Autodesk Fusion 360 part; units mm, degrees
note: some values were not read from the file. Set by a fixed rule: the direction of a hole.
(part 4 of 4)
sketch "草图4" plane through (0, 0, 12) normal (0, 0, 1) x (-1, 0, 0)
  circle A0 centre (-30, 0) radius 1.25
  circle A1 centre (30, 0) radius 1.25
  arc A2 (-16.1674, -6.698) -> (16.1674, -6.698) centre (0, 0) ccw
  arc A3 (18.7154, -4.8546) -> (16.1674, -6.698) centre (18.939, -7.8463) ccw
  line L0 (18.7154, -4.8546) -> (30.2981, -3.9889)
  arc A4 (30.2981, -3.9889) -> (30.2981, 3.9889) centre (30, 0) ccw
  line L1 (30.2981, 3.9889) -> (18.7154, 4.8546)
  arc A5 (16.1674, 6.698) -> (18.7154, 4.8546) centre (18.939, 7.8463) ccw
  arc A6 (16.1674, 6.698) -> (-16.1674, 6.698) centre (0, 0) ccw
  arc A7 (-18.7154, 4.8546) -> (-16.1674, 6.698) centre (-18.939, 7.8463) ccw
  line L2 (-18.7154, 4.8546) -> (-30.2981, 3.9889)
  arc A8 (-30.2981, 3.9889) -> (-30.2981, -3.9889) centre (-30, 0) ccw
  line L3 (-30.2981, -3.9889) -> (-18.7154, -4.8546)
  arc A9 (-16.1674, -6.698) -> (-18.7154, -4.8546) centre (-18.939, -7.8463) ccw
  circle A10 centre (11.6913, 6.75) radius 3
  circle A11 centre (0, -13.5) radius 3
  circle A12 centre (-11.6913, -6.75) radius 3
  circle A13 centre (0, 13.5) radius 3
  circle A14 centre (11.6913, -6.75) radius 3
  circle A15 centre (-11.6913, 6.75) radius 3
  circle A16 centre (0, 0) radius 8
  dimension "d32" = 16
  constraint concentric A2 A16
  measures "d32" diameter of A16
extrude "拉伸7" cut sketch "草图4" against normal up to surface (12 mm away) contours A16 bodies 1

design "J4-J5-Out"
part number: 2026-08-07-17-32-29-090
Autodesk Fusion 360 part; units mm, degrees
sketch "草图1" plane through (0, 0, 0) normal (0, 0, 1) x (1, 0, 0)
  circle A0 centre (0, 0) radius 19
  circle A1 centre (0, 0) radius 25 construction
  arc A2 (-28.5, 0) -> (28.5, 0) centre (0, 0) ccw
  line L0 (-28.5, 0) -> (-28.5, 18)
  line L1 (-28.5, 18) -> (-33.5, 18)
  line L2 (-33.5, 18) -> (-33.5, 58)
  line L3 (-33.5, 58) -> (33.5, 58)
  line L4 (33.5, 58) -> (33.5, 18)
  line L5 (33.5, 18) -> (28.5, 18)
  line L6 (28.5, 18) -> (28.5, 0)
  line L7 (0, 0) -> (0, 58) construction
  circle A3 centre (-12.5, -21.6506) radius 1.6
  circle A4 centre (12.5, -21.6506) radius 1.6
  circle A5 centre (25, 0) radius 1.6
  circle A6 centre (12.5, 21.6506) radius 1.6
  circle A7 centre (-12.5, 21.6506) radius 1.6
  circle A8 centre (-25, 0) radius 1.6
  line L8 (-15, 46) -> (15, 46)
  line L9 (15, 46) -> (15, 33)
  line L10 (15, 33) -> (-15, 33)
  line L11 (-15, 33) -> (-15, 46)
  line L12 (-15, 46) -> (15, 33) construction
  line L13 (15, 46) -> (-15, 33) construction
  point P0 (0, 39.5)
  dimension "d1" = 28.5
  dimension "d2" = 50
  dimension "d3" = 38
  dimension "d4" = 3.2
  dimension "d6" = 360
  dimension "d7" = 67
  dimension "d8" = 40
  dimension "d9" = 58
  dimension "d10" = 13
  dimension "d12" = 30
  dimension "d104" = 12
  constraint coincident A0.centre A1.centre
  constraint concentric A0 A1
  constraint tangent A2 L0
  constraint vertical L0
  constraint perpendicular L0 L1
  constraint perpendicular L1 L2
  constraint perpendicular L2 L3
  constraint perpendicular L3 L4
  constraint perpendicular L4 L5
  constraint perpendicular L5 L6
  constraint tangent A2 L6
  constraint midpoint L3 L7.end
  constraint vertical L7
  constraint equal L2 L4
  constraint coincident A1 A3.centre
  constraint symmetric L7 A3.centre A4.centre
  constraint horizontal L8
  constraint perpendicular L8 L9
  constraint parallel L8 L10
  constraint parallel L9 L11
  constraint coincident L12 P0
  constraint coincident L13 P0
  constraint coincident L7 P0
  measures "d1" radius of A2
  measures "d2" diameter of A1
  measures "d3" diameter of A0
  measures "d4" diameter of A3
  measures "d7" distance of L2.end L3.end
  measures "d8" distance of L1.end L2.end
  measures "d9" distance of A0.centre L3
  measures "d10" distance of L8.start L10.end
  measures "d12" distance of L8.start L8.end
  measures "d104" distance of L3 L8
extrude "拉伸1" add sketch "草图1" along normal blind 5 makes body 1
hole "孔1" at (25, 0, 0) at (12.5, 21.6506, 0) at (-12.5, 21.6506, 0) at (-25, 0, 0) at (-12.5, -21.6506, 0) at (12.5, -21.6506, 0) direction (0, 0, 1) diameter 3.2 depth 10 tip angle 180 countersink diameter 6.3 countersink angle 90 bodies 1
sketch "草图5" plane through (0, 0, 0) normal (0, 0, -1) x (1, 0, 0)
  arc A0 (28.5, 0) -> (-28.5, 0) centre (0, 0) ccw
  line L0 (-28.5, 0) -> (-28.5, -18)
  line L1 (-28.5, -18) -> (-33.5, -18)
  line L2 (-33.5, -18) -> (-33.5, -58)
  line L3 (-33.5, -58) -> (33.5, -58)
  line L4 (33.5, -58) -> (33.5, -18)
  line L5 (33.5, -18) -> (28.5, -18)
  line L6 (28.5, -18) -> (28.5, 0)
  circle A1 centre (0, 0) radius 19
  line L7 (-15, -33) -> (15, -33)
  line L8 (15, -33) -> (15, -46)
  line L9 (15, -46) -> (-15, -46)
  line L10 (-15, -46) -> (-15, -33)
  line L11 (33.5, -18) -> (25.5, -18)
  line L12 (25.5, -18) -> (25.5, -58)
  line L13 (25.5, -58) -> (33.5, -58)
  line L14 (33.5, -58) -> (33.5, -18)
  line L15 (-33.5, -18) -> (-25.5, -18)
  line L16 (-25.5, -18) -> (-25.5, -58)
  line L17 (-25.5, -58) -> (-33.5, -58)
  line L18 (-33.5, -58) -> (-33.5, -18)
  circle A2 centre (12.5, 21.6506) radius 3.15
  circle A3 centre (-25, 0) radius 3.15
  circle A4 centre (12.5, -21.6506) radius 3.15
  circle A5 centre (25, 0) radius 3.15
  circle A6 centre (-12.5, -21.6506) radius 3.15
  circle A7 centre (-12.5, 21.6506) radius 3.15
  dimension "d29" = 8
  constraint horizontal L11
  constraint vertical L12
  constraint horizontal L13
  constraint vertical L14
  constraint coincident L3 L12.end
  constraint coincident L4.end L5.start
  constraint horizontal L15
  constraint vertical L16
  constraint horizontal L17
  constraint vertical L18
  constraint coincident L3 L16.end
  constraint coincident L1.end L2.start
  constraint equal L13 L17
  measures "d29" distance of L12.end L3.end
extrude "拉伸4" add sketch "草图5" along normal blind 3 contours L3 L4 L5 L11 L12 L13 L14 | L1 L2 L3 L15 L16 L17 L18 bodies 1
sketch "草图10" plane through (0, 0, 5) normal (0, 0, 1) x (-1, 0, 0)
  arc A0 (28.5, 0) -> (-28.5, 0) centre (0, 0) ccw
  line L0 (-28.5, 0) -> (-28.5, -18)
  line L1 (-28.5, -18) -> (-33.5, -18)
  line L2 (-33.5, -18) -> (-33.5, -58)
  line L3 (-33.5, -58) -> (33.5, -58)
  line L4 (33.5, -58) -> (33.5, -18)
  line L5 (33.5, -18) -> (28.5, -18)
  line L6 (28.5, -18) -> (28.5, 0)
  circle A1 centre (25, 0) radius 1.6
  line L7 (-15, -33) -> (15, -33)
  line L8 (15, -33) -> (15, -46)
  line L9 (15, -46) -> (-15, -46)
  line L10 (-15, -46) -> (-15, -33)
  circle A2 centre (12.5, -21.6506) radius 1.6
  circle A3 centre (-25, 0) radius 1.6
  circle A4 centre (-12.5, -21.6506) radius 1.6
  circle A5 centre (12.5, 21.6506) radius 1.6
  circle A6 centre (-12.5, 21.6506) radius 1.6
  circle A7 centre (0, 0) radius 19
  line L11 (-20, -33) -> (20, -33) construction
  line L12 (0, 0) -> (0, -33) construction
  circle A8 centre (-20, -33) radius 1.6
  circle A9 centre (20, -33) radius 1.6
  dimension "d78" = 3.2
  dimension "d79" = 40
  dimension "d80" = 33
  constraint perpendicular L8 L11
  constraint coincident A0.centre A7.centre
  constraint midpoint L11 L12.end
  constraint vertical L12
  constraint coincident L11.start A8.centre
  constraint coincident L11.end A9.centre
  constraint equal A8 A9
  measures "d78" diameter of A8
  measures "d79" distance of L11.start L11.end
  measures "d80" distance of A0.centre L12.end
extrude "拉伸10" cut sketch "草图10" against normal up to surface (5 mm away) contours A8 | A9 bodies 1
sketch "草图12" plane through (0, 0, 5) normal (0, 0, 1) x (-1, 0, 0)
  circle A0 centre (-25, 0) radius 1.6
  circle A1 centre (-12.5, 21.6506) radius 1.6
  circle A2 centre (-12.5, -21.6506) radius 1.6
  line L0 (-15, -33) -> (15, -33)
  line L1 (15, -33) -> (15, -46)
  line L2 (15, -46) -> (-15, -46)
  line L3 (-15, -46) -> (-15, -33)
  circle A3 centre (25, 0) radius 1.6
  circle A4 centre (12.5, 21.6506) radius 1.6
  circle A5 centre (12.5, -21.6506) radius 1.6
  circle A6 centre (0, 0) radius 19
  arc A7 (28.5, 0) -> (-28.5, 0) centre (0, 0) ccw
  line L4 (-28.5, 0) -> (-28.5, -18)
  line L5 (-33.5, -18) -> (-33.5, -58)
  line L6 (-33.5, -58) -> (33.5, -58)
  line L7 (33.5, -58) -> (33.5, -18)
  line L8 (28.5, -18) -> (28.5, 0)
  circle A8 centre (20, -33) radius 1.6
  circle A9 centre (-20, -33) radius 1.6
  line L9 (-24, -58) -> (-15, -50)
  line L10 (15, -50) -> (24, -58)
  line L11 (0, 0) -> (0, -58) construction
  line L12 (-15, -50) -> (15, -50)
  line L13 (-28.5, -18) -> (-33.5, -18)
  line L14 (33.5, -18) -> (28.5, -18)
  dimension "d96" = 48
  dimension "d106" = 8
  constraint coincident L6 L9.start
  constraint coincident L3 L9.end
  constraint coincident L1 L10.start
  constraint coincident L6 L10.end
  constraint coincident A6.centre A7.centre
  constraint midpoint L6 L11.end
  constraint symmetric L9.end L10.start L11
  constraint symmetric L9.start L10.end L11
  measures "d96" distance of L9.start L10.end
  measures "d106" distance of L6 L12
extrude "拉伸12" cut sketch "草图12" against normal up to surface (5 mm away) contours L6 L9 L10 L12 bodies 1
fillet "圆角5" radius 2.5 2 edges at (-24, 58, 2.5) (24, 58, 2.5) on bodies 1
fillet "圆角5" radius 3 2 edges at (15, 50, 2.5) (-15, 50, 2.5) on bodies 1
sketch "草图6" plane through (33.5, 0, 0) normal (1, 0, 0) x (0, 1, 0)
  line L0 (58, -3) -> (58, 5)
  line L1 (58, 5) -> (18, 5)
  line L2 (18, 5) -> (18, -3)
  line L3 (18, -3) -> (58, -3)
  line L4 (18, 1) -> (58, 1) construction
  line L5 (38, 5) -> (38, -3) construction
  circle A0 centre (22, 1) radius 1.25
  circle A1 centre (38, 1) radius 1.25
  circle A2 centre (54, 1) radius 1.25
  dimension "d32" = 2.5
  dimension "d33" = 32
  constraint midpoint L2 L4.start
  constraint midpoint L0 L4.end
  constraint coincident L1 L5.start
  constraint coincident L3 L5.end
  constraint perpendicular L3 L5
  constraint midpoint L1 L5.start
  constraint coincident L4 A0.centre
  constraint midpoint L5 A1.centre
  constraint coincident L4 A2.centre
  constraint equal A0 A1
  constraint equal A1 A2
  constraint symmetric L5 A0.centre A2.centre
  measures "d32" diameter of A0
  measures "d33" distance of A0.centre A2.centre
extrude "拉伸5" cut sketch "草图6" against normal blind 6 contours A0 | A1 | A2 bodies 1
mirror "镜像1" about plane through (0, 0, 0) normal (1, 0, 0) of "拉伸5"
fillet "圆角3" radius 5 2 edges at (28.5, 18, 2.5) (-28.5, 18, 2.5) on bodies 1
fillet "圆角3" radius 2 4 edges at (-15, 46, 2.5) (15, 46, 2.5) (15, 33, 2.5) (-15, 33, 2.5) on bodies 1
sketch "草图7" plane through (33.5, 0, 0) normal (1, 0, 0) x (0, 1, 0)
  circle A0 centre (22, 1) radius 1.25
  circle A1 centre (38, 1) radius 1.25
  circle A2 centre (54, 1) radius 1.25
  line L0 (18, 0) -> (18, -3)
  line L1 (18, -3) -> (58, -3)
  circle A3 centre (74, -41) radius 7
  circle A4 centre (74, -41) radius 13.5 construction
  circle A5 centre (63.75, -49.7857) radius 1.6
  line L2 (18, 0) -> (18, -3)
  arc A6 (54.0752, -39.2667) -> (75.3344, -21.0446) centre (74, -41) ccw
  line L3 (74, -41) -> (38, 1) construction
  line L4 (30, -11.1789) -> (54.0752, -39.2667)
  line L5 (75.3344, -21.0446) -> (58, -0.8211)
  circle A7 centre (76.4836, -54.2696) radius 1.6
  circle A8 centre (86.7336, -45.4839) radius 1.6
  circle A9 centre (84.25, -32.2143) radius 1.6
  circle A10 centre (71.5164, -27.7304) radius 1.6
  circle A11 centre (61.2664, -36.5161) radius 1.6
  circle A12 centre (22, 1) radius 1.6
  circle A13 centre (38, 1) radius 1.6
  circle A14 centre (54, 1) radius 1.6
  line L6 (58, 5) -> (18, 5)
  line L7 (58, -3) -> (58, 5)
  line L8 (30, -11.1789) -> (30, -3)
  line L9 (18, -3) -> (30, -3)
  line L10 (18, 5) -> (18, 0)
  dimension "d36" = 41
  dimension "d37" = 74
  dimension "d38" = 27
  dimension "d39" = 14
  dimension "d40" = 3.2
  dimension "d41" = 20
  dimension "d42" = 28
  dimension "d45" = 360
  dimension "d46" = 3.2
  dimension "d77" = 12
  constraint concentric A3 A4
  constraint coincident A4 A5.centre
  constraint coincident L0.start L2.start
  constraint coincident L0.end L1.start
  constraint coincident A3.centre A4.centre
  constraint coincident A1.centre L3.end
  constraint symmetric A6.start A6.end L3
  constraint parallel L4 L5
  constraint parallel L3 L4
  constraint symmetric L3 A10.centre A11.centre
  constraint concentric A0 A12
  constraint concentric A2 A14
  constraint equal A12 A13
  constraint equal A13 A14
  constraint coincident L1 L8.end
  constraint perpendicular L1 L8
  constraint coincident L5.end L7
  measures "d36" vertical distance of origin A3.centre
  measures "d37" horizontal distance of origin A3.centre
  measures "d38" diameter of A4
  measures "d39" diameter of A3
  measures "d40" diameter of A5
  measures "d41" radius of A6
  measures "d42" distance of L4 L5
  measures "d46" diameter of A12
  measures "d77" distance of L2 L8
extrude "拉伸6" add sketch "草图7" along normal blind 4 separate body contours L0 L1 L2 L6 L7 L9 L10 | L1 A6 L4 L5 L7 L8 | A5 | A7 | A8 | A9 | A10 | A11 makes body 2
sketch "草图8" plane through (37.5, 0, 0) normal (1, 0, 0) x (0, 1, 0)
  line L0 (58, -0.8211) -> (58, 5)
  line L1 (54.3615, -9) -> (65.6291, -22.2707)
  line L2 (65.6291, -22.2707) -> (56.4816, -30.0375)
  line L3 (56.4816, -30.0375) -> (38.6196, -9)
  line L4 (74, -41.4) -> (61.0554, -26.1541) construction
  line L5 (54.3615, -9) -> (38.6196, -9)
  line L6 (18, -3) -> (30, -3)
  circle A0 centre (74, -41) radius 7
  arc A1 (54.0752, -39.2667) -> (75.3344, -21.0446) centre (74, -41) ccw
  line L7 (75.3344, -21.0446) -> (58, -0.8211)
  line L8 (30, -3) -> (30, -11.1789)
  line L9 (30, -11.1789) -> (54.0752, -39.2667)
  circle A2 centre (38, 1) radius 1.6
  circle A3 centre (22, 1) radius 1.6
  circle A4 centre (54, 1) radius 1.6
  line L10 (58, 5) -> (18, 5)
  line L11 (18, 5) -> (18, -3)
  dimension "d51" = 20
  dimension "d53" = 12
  constraint perpendicular L1 L2
  constraint perpendicular L2 L3
  constraint midpoint L2 L4.end
  constraint horizontal L5
  measures "d51" distance of L2 L4.start
  measures "d53" distance of L1.end L2.end
extrude "拉伸7" cut sketch "草图8" against normal up to surface (4 mm away) contours L1 L2 L3 L5 bodies 2
fillet "圆角2" radius 2 4 edges at (35.5, 38.6196, -9) (35.5, 65.6291, -22.2707) (35.5, 56.4816, -30.0375) (35.5, 30, -3) on bodies 2
fillet "圆角2" radius 8 2 edges at (35.5, 54.3615, -9) (35.5, 58, -0.8211) on bodies 2
fillet "圆角2" radius 8 3 edges at (35.5, 75.3344, -21.0446) (35.5, 54.0752, -39.2667) (35.5, 30, -11.1789) on bodies 2
fillet "圆角2" radius 0.8 3 edges at (35.5, 18, 5) (35.5, 18, -3) (35.5, 58, 5) on bodies 2
mirror "镜像2" about plane through (0, 0, 0) normal (1, 0, 0) of "拉伸6", "拉伸7", "圆角2" makes body 3
extrude "拉伸8" cut sketch "草图7" along normal up to surface (4 mm away) contours A5 | A7 | A8 | A9 | A10 | A11 bodies 2
sketch "草图9" plane through (-37.5, 0, 0) normal (-1, 0, 0) x (0, -1, 0)
  line L0 (-74, -41.4) -> (-86.9446, -56.6459) construction
  circle A0 centre (-74, -41.4) radius 13 construction
  circle A1 centre (-86.2416, -45.7752) radius 1.6
  circle A2 centre (-76.3318, -54.1892) radius 1.6
  circle A3 centre (-64.0902, -49.814) radius 1.6
  circle A4 centre (-61.7584, -37.0248) radius 1.6
  circle A5 centre (-71.6682, -28.6108) radius 1.6
  circle A6 centre (-83.9098, -32.986) radius 1.6
  line L1 (-28, -3) -> (-18.8, -3)
  arc A7 (-31.9259, -13.4259) -> (-30, -8.2195) centre (-38, -8.2195) ccw
  line L2 (-30, -8.2195) -> (-30, -5)
  arc A8 (-28, -3) -> (-30, -5) centre (-28, -5) ccw
  arc A9 (-59.9259, -3.068) -> (-58, 2.1383) centre (-66, 2.1383) ccw
  line L3 (-59.9259, -3.068) -> (-73.3576, -18.7382)
  arc A10 (-77.8797, -21.3799) -> (-73.3576, -18.7382) centre (-79.4316, -13.5319) ccw
  arc A11 (-77.8797, -21.3799) -> (-54.0174, -41.8334) centre (-74, -41) ccw
  arc A12 (-52.0984, -36.9604) -> (-54.0174, -41.8334) centre (-46.0243, -42.1667) ccw
  line L4 (-52.0984, -36.9604) -> (-31.9259, -13.4259)
  line L5 (-58.0062, -28.743) -> (-64.1046, -23.5652)
  arc A13 (-64.3347, -20.7461) -> (-64.1046, -23.5652) centre (-62.8101, -22.0406) ccw
  line L6 (-64.3347, -20.7461) -> (-56.7577, -11.8222)
  arc A14 (-50.6594, -9) -> (-56.7577, -11.8222) centre (-50.6594, -17) ccw
  line L7 (-50.6594, -9) -> (-42.9414, -9)
  arc A15 (-41.4168, -12.2945) -> (-42.9414, -9) centre (-42.9414, -11) ccw
  line L8 (-41.4168, -12.2945) -> (-55.1872, -28.5129)
  arc A16 (-58.0062, -28.743) -> (-55.1872, -28.5129) centre (-56.7117, -27.2185) ccw
  circle A17 centre (-74, -41) radius 7
  line L9 (-18, -2.2) -> (-18, 4.2)
  line L10 (-18.8, 5) -> (-57.2, 5)
  line L11 (-58, 4.2) -> (-58, 2.1383)
  circle A18 centre (-54, 1) radius 1.6
  circle A19 centre (-22, 1) radius 1.6
  circle A20 centre (-38, 1) radius 1.6
  arc A21 (-18.8, -3) -> (-18, -2.2) centre (-18.8, -2.2) ccw
  arc A22 (-18, 4.2) -> (-18.8, 5) centre (-18.8, 4.2) ccw
  arc A23 (-57.2, 5) -> (-58, 4.2) centre (-57.2, 4.2) ccw
  dimension "d67" = 3.2
  dimension "d69" = 360
  dimension "d70" = 26
  constraint coincident L0.start A0.centre
  constraint coincident A0 A1.centre
  constraint symmetric L0 A1.centre A2.centre
  measures "d67" diameter of A1
  measures "d70" diameter of A0
extrude "拉伸9" cut sketch "草图9" against normal up to surface (4 mm away) contours A1 | A2 | A3 | A4 | A5 | A6 bodies 3
sketch "草图11" plane through (0, 0, 0) normal (0, 0, -1) x (1, 0, 0)
  circle A0 centre (0, 0) radius 19
  arc A1 (15, -35) -> (13, -33) centre (13, -35) ccw
  line L0 (15, -35) -> (15, -44)
  arc A2 (13, -46) -> (15, -44) centre (13, -44) ccw
  line L1 (13, -46) -> (-13, -46)
  arc A3 (-15, -44) -> (-13, -46) centre (-13, -44) ccw
  line L2 (-15, -44) -> (-15, -35)
  arc A4 (-13, -33) -> (-15, -35) centre (-13, -35) ccw
  line L3 (-13, -33) -> (13, -33)
  line L4 (-33.5, -18) -> (-25.5, -18)
  line L5 (-25.5, -18) -> (-25.5, -58)
  line L6 (24.9505, -58) -> (25.5, -58)
  line L7 (25.5, -58) -> (25.5, -18)
  line L8 (25.5, -18) -> (33.5, -18)
  arc A5 (28.5, -13) -> (33.5, -18) centre (33.5, -13) ccw
  line L9 (28.5, -13) -> (28.5, 0)
  arc A6 (28.5, 0) -> (-28.5, 0) centre (0, 0) ccw
  line L10 (-28.5, 0) -> (-28.5, -13)
  arc A7 (-33.5, -18) -> (-28.5, -13) centre (-33.5, -13) ccw
  circle A8 centre (-20, -33) radius 1.6
  circle A9 centre (20, -33) radius 1.6
  circle A10 centre (20, -33) radius 1.25
  circle A11 centre (-20, -33) radius 1.25
  line L11 (25, -28.5) -> (-25, -28.5)
  line L12 (-25, -28.5) -> (-25, -37.5)
  line L13 (-25, -37.5) -> (-15, -37.5)
  line L14 (-15, -37.5) -> (-15, -33)
  line L15 (-15, -33) -> (15, -33)
  line L16 (15, -33) -> (15, -37.5)
  line L17 (15, -37.5) -> (25, -37.5)
  line L18 (25, -37.5) -> (25, -28.5)
  line L19 (0, 0) -> (0, -28.5) construction
  line L20 (20, -33) -> (20, -37.5) construction
  circle A12 centre (-12.5, 21.6506) radius 3.15
  circle A13 centre (-12.5, -21.6506) radius 3.15
  circle A14 centre (25, 0) radius 3.15
  circle A15 centre (12.5, -21.6506) radius 3.15
  circle A16 centre (-25, 0) radius 3.15
  circle A17 centre (12.5, 21.6506) radius 3.15
  arc A18 (23.2896, -57.3685) -> (24.9505, -58) centre (24.9505, -55.5) ccw
  line L21 (-25.5, -58) -> (-24.9505, -58)
  arc A19 (-24.9505, -58) -> (-23.2896, -57.3685) centre (-24.9505, -55.5) ccw
  line L22 (-23.2896, -57.3685) -> (-15.8525, -50.7578)
  arc A20 (-13.8594, -50) -> (-15.8525, -50.7578) centre (-13.8594, -53) ccw
  line L23 (-13.8594, -50) -> (13.8594, -50)
  arc A21 (15.8525, -50.7578) -> (13.8594, -50) centre (13.8594, -53) ccw
  line L24 (15.8525, -50.7578) -> (23.2896, -57.3685)
  dimension "d83" = 2.5
  dimension "d84" = 4.5
  dimension "d85" = 10
  dimension "d86" = 9
  constraint concentric A9 A10
  constraint concentric A8 A11
  constraint equal A10 A11
  constraint horizontal L11
  constraint perpendicular L11 L12
  constraint perpendicular L12 L13
  constraint perpendicular L13 L14
  constraint perpendicular L14 L15
  constraint perpendicular L15 L16
  constraint perpendicular L16 L17
  constraint perpendicular L11 L18
  constraint midpoint L11 L19.end
  constraint vertical L19
  constraint coincident A0.centre A6.centre
  constraint symmetric L14.end L15.end L19
  constraint symmetric L12.end L17.end L19
  constraint coincident A9.centre A10.centre
  constraint midpoint L17 L20.end
  constraint vertical L20
  constraint collinear L3 L15
  measures "d83" diameter of A10
  measures "d84" distance of L3 L11
  measures "d85" distance of L16.end L17.end
  measures "d86" distance of L11.start L17.end
extrude "拉伸11" add sketch "草图11" along normal blind 8 separate body contours L0 L2 L3 L11 L12 L13 L14 L15 L16 L17 L18 | A8 | A9 makes body 4
fillet "圆角4" radius 2 8 edges at (15, 33, -4) (-15, 33, -4) (-15, 37.5, -4) (15, 37.5, -4) (25, 37.5, -4) (25, 28.5, -4) (-25, 28.5, -4) (-25, 37.5, -4) on bodies 4
equation "d1 = ( 57 / 2 ) * 1 mm"

design "yawτö╡µ£║σ¢║σ«Üµ¥┐"
part number: 2026-08-10-17-08-21-834
Autodesk Fusion 360 part; units mm, degrees
sketch "草图1" plane through (0, 0, 0) normal (0, 1, 0) x (1, 0, 0)
  circle A0 centre (0, 0) radius 20
  circle A1 centre (0, 0) radius 25 construction
  circle A2 centre (0, 25) radius 1.65
  circle A3 centre (-21.6506, 12.5) radius 1.65
  circle A4 centre (-21.6506, -12.5) radius 1.65
  circle A5 centre (0, -25) radius 1.65
  circle A6 centre (21.6506, -12.5) radius 1.65
  circle A7 centre (21.6506, 12.5) radius 1.65
  line L0 (45, -15) -> (-45, -15)
  line L1 (-45, -15) -> (-45, 15)
  line L2 (-45, 15) -> (45, 15)
  line L3 (45, 15) -> (45, -15)
  line L4 (45, -15) -> (-45, 15) construction
  line L5 (-45, -15) -> (45, 15) construction
  circle A8 centre (0, 0) radius 30
  dimension "d1" = 40
  dimension "d2" = 3.3
  dimension "d4" = 360
  dimension "d5" = 50
  dimension "d24" = 30
  dimension "d25" = 60
  dimension "d26" = 90
  constraint coincident A0.centre A1.centre
  constraint coincident A1 A2.centre
  constraint vertical A2.centre A5.centre
  constraint horizontal L0
  constraint perpendicular L0 L1
  constraint parallel L0 L2
  constraint parallel L1 L3
  constraint coincident L4 A0.centre
  constraint coincident L5 A0.centre
  measures "d1" diameter of A0
  measures "d2" diameter of A2
  measures "d5" diameter of A1
  measures "d24" distance of L0.start L2.end
  measures "d25" diameter of A8
  measures "d26" distance of L1.end L2.end
extrude "拉伸1" add sketch "草图1" along normal blind 3 contours A0 L0 L2 A8 | A0 L2 A8 | A0 L0 A8 | A0 L0 L2 A8 | L0 L2 L3 A8 | L0 L1 L2 A8
chamfer "倒角3" distance 3 angle 45 4 edges at (45, 1.5, -15) (45, 1.5, 15) (-45, 1.5, -15) (-45, 1.5, 15)
sketch "草图5" plane through (0, 3, 0) normal (0, 1, 0) x (-1, 0, 0)
  line L0 (45, 12) -> (42, 15)
  line L1 (42, 15) -> (25.9808, 15)
  arc A0 (25.9808, 15) -> (-25.9808, 15) centre (0, 0) ccw
  line L2 (-25.9808, 15) -> (-42, 15)
  line L3 (-42, 15) -> (-45, 12)
  line L4 (-45, 12) -> (-45, -12)
  line L5 (-45, -12) -> (-42, -15)
  line L6 (-42, -15) -> (-25.9808, -15)
  arc A1 (-25.9808, -15) -> (25.9808, -15) centre (0, 0) ccw
  line L7 (25.9808, -15) -> (42, -15)
  line L8 (42, -15) -> (45, -12)
  line L9 (45, -12) -> (45, 12)
  circle A2 centre (0, 0) radius 20
  circle A3 centre (0, 25) radius 1.65
  circle A4 centre (-21.6506, 12.5) radius 1.65
  circle A5 centre (0, -25) radius 1.65
  circle A6 centre (21.6506, -12.5) radius 1.65
  circle A7 centre (-21.6506, -12.5) radius 1.65
  circle A8 centre (21.6506, 12.5) radius 1.65
  circle A9 centre (-41, 10) radius 1.65
  circle A10 centre (-41, -10) radius 1.65
  line L10 (0, 0) -> (0, 37.6394) construction
  circle A11 centre (41, 10) radius 1.65
  circle A12 centre (41, -10) radius 1.65
  dimension "d31" = 3.3
  dimension "d32" = 5
  dimension "d33" = 4
  dimension "d36" = 0
  dimension "d37" = -20
  constraint coincident A0.centre A1.centre
  constraint perpendicular L2 L10
  constraint symmetric A9 L10 A11
  constraint symmetric A10 L10 A12
  measures "d31" diameter of A9
  measures "d32" distance of L2 A9.centre
  measures "d33" distance of L4 A9.centre
extrude "拉伸5" cut sketch "草图5" against normal blind 26 contours A9 | A10 | A11 | A12
sketch "草图7" plane through (0, 0, 0) normal (0, -1, 0) x (1, 0, 0)
  line L0 (-42, 15) -> (-45, 12)
  line L1 (-45, 12) -> (-45, -12)
  line L2 (-45, -12) -> (-42, -15)
  line L3 (-42, -15) -> (-25.9808, -15)
  arc A0 (-25.9808, -15) -> (25.9808, -15) centre (0, 0) ccw
  line L4 (25.9808, -15) -> (42, -15)
  line L5 (42, -15) -> (45, -12)
  line L6 (45, -12) -> (45, 12)
  line L7 (45, 12) -> (42, 15)
  line L8 (42, 15) -> (25.9808, 15)
  arc A1 (25.9808, 15) -> (-25.9808, 15) centre (0, 0) ccw
  line L9 (-25.9808, 15) -> (-42, 15)
  circle A2 centre (0, 0) radius 20
  circle A3 centre (0, -25) radius 1.65
  circle A4 centre (21.6506, 12.5) radius 1.65
  circle A5 centre (0, 25) radius 1.65
  circle A6 centre (-21.6506, 12.5) radius 1.65
  circle A7 centre (21.6506, -12.5) radius 1.65
  circle A8 centre (-21.6506, -12.5) radius 1.65
  circle A9 centre (-41, -10) radius 1.65
  circle A10 centre (41, 10) radius 1.65
  circle A11 centre (-41, 10) radius 1.65
  circle A12 centre (41, -10) radius 1.65
hole "孔3" at (-41, 0, 10) at (-41, 0, -10) at (41, 0, 10) at (41, 0, -10) direction (0, 1, 0) diameter 3.3 depth 8 tip angle 180 countersink diameter 6.3 countersink angle 90
